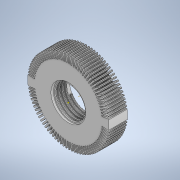
# Autodesk Inventor part: Scheibe
Saved by Autodesk Inventor 2020 (Build 240168000, 168)
## iProperties
Created: 2019-06-20
Part Number: Scheibe
Material: Generisch
Document SubType Name: Modeling
Designer: Limmer
Density: 1 g/cm^3
Appearance: Vorgabe
Author: Limmer
Autodesk Inventor part; units mm, degrees
(part 1 of 2)
ref_plane "YZ Plane" through (0, 0, 0) normal (1, 0, 0) x (0, 1, 0)
ref_plane "XZ Plane" through (0, 0, 0) normal (0, 1, 0) x (-1, 0, 0)
ref_plane "XY Plane" through (0, 0, 0) normal (0, 0, 1) x (1, 0, 0)
sketch "Skizze1" plane through (0, 0, 0) normal (0, 0, 1) x (1, 0, 0)
  circle A0 centre (0, 0) radius 17.5
  circle A1 centre (0, 0) radius 7.5
  dimension "d0" = 35
  dimension "d1" = 15
  constraints: 2 centre point, 2 coincident
  measures "d0" diameter of A0
  measures "d1" diameter of A1
extrude "Extrusion1" add sketch "Skizze1" along normal blind 8
sketch "Skizze2" plane through (0, 0, 0) normal (1, 0, 0) x (0, 1, 0)
  line L0 (-7.5, 0) -> (7.5, 0) projected
  line L1 (-7.5, 8) -> (7.5, 8) projected
  line L2 (7.5, 8) -> (6.75, 8)
  line L3 (6.75, 8) -> (6.75, 7.25)
  line L4 (6.75, 7.25) -> (7.5, 7.25)
  line L5 (7.5, 7.25) -> (7.5, 8)
  point P0 (0, 0)
  dimension "d4" = 0.75
  dimension "d5" = 0.75
  constraints: 8 end point, 2 parallel, 1 horizontal, 1 perpendicular
  measures "d4" distance of L4.end L3.end
  measures "d5" distance of L3.end L2.end
coil "Spirale1" sketch "Skizze2" operation add axis through (0, 0, 0) along (0, 0, -1) pitch 1.5 turns 4.666667 hand right
fillet "Rundung1" radius 0.25 20 edges at (2.7455, -6.1664, 1.35) (6.713, 0.7056, 7.65) (5.8457, 3.375, 6.25) (-6.4196, -2.0859, 6.95) (-1.4034, 6.6025, 2.05) (0, -6.75, 2.75) (1.4034, 6.6025, 3.45) (-5.0162, -4.5166, 5.55) (3.9676, 5.4609, 4.85) (-2.7455, -6.1664, 4.15) (2.7455, -6.1664, 0.6) (1.4034, 6.6025, 2.7) (0, -6.75, 2) (-1.4034, 6.6025, 1.3) (6.713, 0.7056, 6.9) (3.9676, 5.4609, 4.1) (-2.7455, -6.1664, 3.4) (5.8457, 3.375, 5.5) (-6.4196, -2.0859, 6.2) (-5.0162, -4.5166, 4.8)
fillet "Rundung2" radius 0.25 10 edges at (0, 6.75, 7.625) (0, 6.8232, 7.3233) (0, 7.25, 7.25) (0, 7.25, 8) (0, 6.8232, 7.9267) (-6.2787, -3.625, 1) (-5.8457, -3.375, 0.625) (-5.9091, -3.4116, 0.3233) (-6.2787, -3.625, 0.25) (-5.9091, -3.4116, 0.9267)
sketch "Skizze4" plane through (0, 0, 8) normal (0, 0, 1) x (1, 0, 0)
  point P0 (0, 0)
sketch "Skizze5" plane through (0, 0, 8) normal (0, 0, 1) x (1, 0, 0)
  circle A0 centre (0, 0) radius 17.5 projected
  line L0 (0, -17.2583) -> (0, -14.738)
  line L1 (0, 0) -> (-0.506, -14.4912) construction
  line L2 (0, 0) -> (0, -17) construction
  arc A1 (0.2433, -17.4983) -> (0.3675, -17.4961) centre (0, 0) ccw
  line L3 (0.5147, -14.7379) -> (0.6023, -17.2478) construction
  line L4 (0, 0) -> (0, -17.5) construction
  line L5 (0.5147, -14.7379) -> (0.6023, -17.2478)
  arc A2 (0.7422, -14.4898) -> (0.7764, -14.488) centre (0, 0) ccw
  line L6 (0, 0) -> (1.0121, -14.4735) construction
  line L7 (0, 0) -> (0.5064, -14.5) construction
  arc A3 (0, -17.2583) -> (0.2433, -17.4983) centre (0.24, -17.2583) ccw
  arc A4 (0.3675, -17.4961) -> (0.6023, -17.2478) centre (0.3625, -17.2562) ccw
  arc A5 (0.7422, -14.4898) -> (0.5147, -14.7379) centre (0.7545, -14.7295) ccw
  arc A6 (1.0287, -14.711) -> (0.7764, -14.488) centre (0.7893, -14.7277) ccw
  arc A7 (1.2039, -17.2163) -> (1.4634, -17.4387) centre (1.4433, -17.1995) ccw
  arc A8 (1.4634, -17.4387) -> (1.5871, -17.4279) centre (0, 0) ccw
  arc A9 (1.5871, -17.4279) -> (1.804, -17.1638) centre (1.5653, -17.1889) ccw
  arc A10 (1.7512, -14.4028) -> (1.5415, -14.6661) centre (1.7802, -14.641) ccw
  line L8 (1.5415, -14.6661) -> (1.804, -17.1638)
  arc A11 (2.0524, -14.6034) -> (1.7852, -14.3986) centre (1.8147, -14.6368) ccw
  arc A12 (1.7512, -14.4028) -> (1.7852, -14.3986) centre (0, 0) ccw
  line L9 (0, 0) -> (1.2207, -17.4574) construction
  line L10 (1.2039, -17.2163) -> (1.0281, -14.7021)
  arc A13 (2.4019, -17.0904) -> (2.6763, -17.2941) centre (2.6396, -17.057) ccw
  arc A14 (2.6763, -17.2941) -> (2.7989, -17.2747) centre (0, 0) ccw
  arc A15 (2.7989, -17.2747) -> (2.9969, -16.9961) centre (2.7605, -17.0378) ccw
  arc A16 (2.7516, -14.2455) -> (2.5608, -14.5228) centre (2.7971, -14.4812) ccw
  line L11 (2.5608, -14.5228) -> (2.9969, -16.9961)
  arc A17 (3.066, -14.4246) -> (2.7852, -14.239) centre (2.8313, -14.4745) ccw
  arc A18 (2.7516, -14.2455) -> (2.7852, -14.239) centre (0, 0) ccw
  line L12 (0, 0) -> (2.4355, -17.3297) construction
  line L13 (2.4019, -17.0904) -> (2.0511, -14.5946)
  arc A19 (3.5882, -16.8812) -> (3.8761, -17.0653) centre (3.823, -16.8313) ccw
  arc A20 (3.8761, -17.0653) -> (3.9971, -17.0374) centre (0, 0) ccw
  arc A21 (3.9971, -17.0374) -> (4.1752, -16.7457) centre (3.9423, -16.8037) ccw
  arc A22 (3.7386, -14.0189) -> (3.5676, -14.3088) centre (3.8005, -14.2508) ccw
  line L14 (3.5676, -14.3088) -> (4.1752, -16.7457)
  arc A23 (4.0648, -14.1756) -> (3.7717, -14.01) centre (3.8341, -14.2418) ccw
  arc A24 (3.7386, -14.0189) -> (3.7717, -14.01) centre (0, 0) ccw
  line L15 (0, 0) -> (3.6385, -17.1176) construction
  line L16 (3.5882, -16.8812) -> (3.0642, -14.416)
  arc A25 (4.757, -16.5898) -> (5.0571, -16.7534) centre (4.9877, -16.5236) ccw
  arc A26 (5.0571, -16.7534) -> (5.1758, -16.7171) centre (0, 0) ccw
  arc A27 (5.1758, -16.7171) -> (5.3331, -16.4136) centre (5.1049, -16.4878) ccw
  arc A28 (4.7074, -13.7239) -> (4.557, -14.0251) centre (4.7853, -13.951) ccw
  line L17 (4.557, -14.0251) -> (5.3331, -16.4136)
  arc A29 (5.0437, -13.8575) -> (4.7398, -13.7128) centre (4.8182, -13.9396) ccw
  arc A30 (4.7074, -13.7239) -> (4.7398, -13.7128) centre (0, 0) ccw
  line L18 (0, 0) -> (4.8237, -16.8221) construction
  line L19 (4.757, -16.5898) -> (4.0624, -14.1671)
  arc A31 (5.9027, -16.2175) -> (6.2134, -16.3598) centre (6.1282, -16.1354) ccw
  arc A32 (6.2134, -16.3598) -> (6.3294, -16.3153) centre (0, 0) ccw
  arc A33 (6.3294, -16.3153) -> (6.4651, -16.0016) centre (6.2426, -16.0916) ccw
  arc A34 (5.6533, -13.3621) -> (5.5243, -13.6731) centre (5.7468, -13.5832) ccw
  line L20 (5.5243, -13.6731) -> (6.4651, -16.0016)
  arc A35 (5.9981, -13.472) -> (5.6848, -13.3488) centre (5.7788, -13.5696) ccw
  arc A36 (5.6533, -13.3621) -> (5.6848, -13.3488) centre (0, 0) ccw
  line L21 (0, 0) -> (5.9854, -16.4446) construction
  line L22 (5.9027, -16.2175) -> (5.0407, -13.8492)
  arc A37 (7.0196, -15.7663) -> (7.3395, -15.8865) centre (7.2388, -15.6687) ccw
  arc A38 (7.3395, -15.8865) -> (7.452, -15.834) centre (0, 0) ccw
  arc A39 (7.452, -15.834) -> (7.5656, -15.5117) centre (7.3498, -15.6169) ccw
  arc A40 (6.5716, -12.9352) -> (6.4646, -13.2544) centre (6.6803, -13.1492) ccw
  line L23 (6.4646, -13.2544) -> (7.5656, -15.5117)
  arc A41 (6.9232, -13.0207) -> (6.6021, -12.9197) centre (6.7113, -13.1334) ccw
  arc A42 (6.5716, -12.9352) -> (6.6021, -12.9197) centre (0, 0) ccw
  line L24 (0, 0) -> (7.1179, -15.987) construction
  line L25 (7.0196, -15.7663) -> (5.9945, -13.4639)
  arc A43 (8.1023, -15.2382) -> (8.4298, -15.3358) centre (8.3142, -15.1255) ccw
  arc A44 (8.4298, -15.3358) -> (8.5384, -15.2756) centre (0, 0) ccw
  arc A45 (8.5384, -15.2756) -> (8.6292, -14.9462) centre (8.4213, -15.0662) ccw
  arc A46 (7.4579, -12.4453) -> (7.3734, -12.7712) centre (7.5813, -12.6512) ccw
  line L26 (7.3734, -12.7712) -> (8.6292, -14.9462)
  arc A47 (7.8147, -12.5061) -> (7.4873, -12.4277) centre (7.6111, -12.6332) ccw
  arc A48 (7.4579, -12.4453) -> (7.4873, -12.4277) centre (0, 0) ccw
  line L27 (0, 0) -> (8.2158, -15.4516) construction
  line L28 (8.1023, -15.2382) -> (6.9191, -13.0129)
  arc A49 (9.1455, -14.6359) -> (9.4791, -14.7105) centre (9.3491, -14.5087) ccw
  arc A50 (9.4791, -14.7105) -> (9.5832, -14.6428) centre (0, 0) ccw
  arc A51 (9.5832, -14.6428) -> (9.6507, -14.3078) centre (9.4518, -14.442) ccw
  arc A52 (8.3079, -11.8948) -> (8.2464, -12.2257) centre (8.4453, -12.0915) ccw
  line L29 (8.2464, -12.2257) -> (9.6507, -14.3078)
  arc A53 (8.668, -11.9305) -> (8.3359, -11.8751) centre (8.4738, -12.0715) ccw
  arc A54 (8.3079, -11.8948) -> (8.3359, -11.8751) centre (0, 0) ccw
  line L30 (0, 0) -> (9.2736, -14.8408) construction
  line L31 (9.1455, -14.6359) -> (7.81, -12.4986)
  arc A55 (10.1442, -13.9623) -> (10.4821, -14.0134) centre (10.3384, -13.8212) ccw
  arc A56 (10.4821, -14.0134) -> (10.5813, -13.9387) centre (0, 0) ccw
  arc A57 (10.5813, -13.9387) -> (10.6253, -13.5998) centre (10.4362, -13.7475) ccw
  arc A58 (9.1174, -11.2863) -> (9.0791, -11.6207) centre (9.2682, -11.4729) ccw
  line L32 (9.0791, -11.6207) -> (10.6253, -13.5998)
  arc A59 (9.4791, -11.2968) -> (9.144, -11.2647) centre (9.2953, -11.451) ccw
  arc A60 (9.1174, -11.2863) -> (9.144, -11.2647) centre (0, 0) ccw
  line L33 (0, 0) -> (10.2862, -14.1578) construction
  line L34 (10.1442, -13.9623) -> (8.6628, -11.9233)
  arc A61 (11.0934, -13.2206) -> (11.4341, -13.2481) centre (11.2773, -13.0664) ccw
  arc A62 (11.4341, -13.2481) -> (11.5278, -13.1666) centre (0, 0) ccw
  arc A63 (11.5278, -13.1666) -> (11.5481, -12.8254) centre (11.3697, -12.986) ccw
  arc A64 (9.8825, -10.6228) -> (9.8676, -10.9591) centre (10.0459, -10.7985) ccw
  line L35 (9.8676, -10.9591) -> (11.5481, -12.8254)
  arc A65 (10.244, -10.608) -> (9.9075, -10.5994) centre (10.0714, -10.7747) ccw
  arc A66 (9.8825, -10.6228) -> (9.9075, -10.5994) centre (0, 0) ccw
  line L36 (0, 0) -> (11.2488, -13.4058) construction
  line L37 (11.0934, -13.2206) -> (9.4734, -11.29)
  arc A67 (11.9886, -12.4146) -> (12.3304, -12.4182) centre (12.1613, -12.2479) ccw
  arc A68 (12.3304, -12.4182) -> (12.4182, -12.3304) centre (0, 0) ccw
  arc A69 (12.4182, -12.3304) -> (12.4146, -11.9886) centre (12.2479, -12.1613) ccw
  arc A70 (10.5994, -9.9075) -> (10.608, -10.244) centre (10.7747, -10.0714) ccw
  line L38 (10.608, -10.244) -> (12.4146, -11.9886)
  arc A71 (10.9591, -9.8676) -> (10.6228, -9.8825) centre (10.7985, -10.0459) ccw
  arc A72 (10.5994, -9.9075) -> (10.6228, -9.8825) centre (0, 0) ccw
  line L39 (0, 0) -> (12.1565, -12.5884) construction
  line L40 (11.9886, -12.4146) -> (10.2379, -10.6017)
  arc A73 (12.8254, -11.5481) -> (13.1666, -11.5278) centre (12.986, -11.3697) ccw
  arc A74 (13.1666, -11.5278) -> (13.2481, -11.4341) centre (0, 0) ccw
  arc A75 (13.2481, -11.4341) -> (13.2206, -11.0934) centre (13.0664, -11.2773) ccw
  arc A76 (11.2647, -9.144) -> (11.2968, -9.4791) centre (11.451, -9.2953) ccw
  line L41 (11.2968, -9.4791) -> (13.2206, -11.0934)
  arc A77 (11.6207, -9.0791) -> (11.2863, -9.1174) centre (11.4729, -9.2682) ccw
  arc A78 (11.2647, -9.144) -> (11.2863, -9.1174) centre (0, 0) ccw
  line L42 (0, 0) -> (13.005, -11.7098) construction
  line L43 (12.8254, -11.5481) -> (10.9525, -9.8617)
  arc A79 (13.5998, -10.6253) -> (13.9387, -10.5813) centre (13.7475, -10.4362) ccw
  arc A80 (13.9387, -10.5813) -> (14.0134, -10.4821) centre (0, 0) ccw
  arc A81 (14.0134, -10.4821) -> (13.9623, -10.1442) centre (13.8212, -10.3384) ccw
  arc A82 (11.8751, -8.3359) -> (11.9305, -8.668) centre (12.0715, -8.4738) ccw
  line L44 (11.9305, -8.668) -> (13.9623, -10.1442)
  arc A83 (12.2257, -8.2464) -> (11.8948, -8.3079) centre (12.0915, -8.4453) ccw
  arc A84 (11.8751, -8.3359) -> (11.8948, -8.3079) centre (0, 0) ccw
  line L45 (0, 0) -> (13.7902, -10.7741) construction
  line L46 (13.5998, -10.6253) -> (11.6137, -9.0736)
  arc A85 (14.3078, -9.6507) -> (14.6428, -9.5832) centre (14.442, -9.4518) ccw
  arc A86 (14.6428, -9.5832) -> (14.7105, -9.4791) centre (0, 0) ccw
  arc A87 (14.7105, -9.4791) -> (14.6359, -9.1455) centre (14.5087, -9.3491) ccw
  arc A88 (12.4277, -7.4873) -> (12.5061, -7.8147) centre (12.6332, -7.6111) ccw
  line L47 (12.5061, -7.8147) -> (14.6359, -9.1455)
  arc A89 (12.7712, -7.3734) -> (12.4453, -7.4579) centre (12.6512, -7.5813) ccw
  arc A90 (12.4277, -7.4873) -> (12.4453, -7.4579) centre (0, 0) ccw
  line L48 (0, 0) -> (14.5082, -9.7859) construction
  line L49 (14.3078, -9.6507) -> (12.2184, -8.2414)
  arc A91 (14.9462, -8.6292) -> (15.2756, -8.5384) centre (15.0662, -8.4213) ccw
  arc A92 (15.2756, -8.5384) -> (15.3358, -8.4298) centre (0, 0) ccw
  arc A93 (15.3358, -8.4298) -> (15.2382, -8.1023) centre (15.1255, -8.3142) ccw
  arc A94 (12.9197, -6.6021) -> (13.0207, -6.9232) centre (13.1334, -6.7113) ccw
  line L50 (13.0207, -6.9232) -> (15.2382, -8.1023)
  arc A95 (13.2544, -6.4646) -> (12.9352, -6.5716) centre (13.1492, -6.6803) ccw
  arc A96 (12.9197, -6.6021) -> (12.9352, -6.5716) centre (0, 0) ccw
  line L51 (0, 0) -> (15.1554, -8.75) construction
  line L52 (14.9462, -8.6292) -> (12.7635, -7.369)
  arc A97 (15.5117, -7.5656) -> (15.834, -7.452) centre (15.6169, -7.3498) ccw
  arc A98 (15.834, -7.452) -> (15.8865, -7.3395) centre (0, 0) ccw
  arc A99 (15.8865, -7.3395) -> (15.7663, -7.0196) centre (15.6687, -7.2388) ccw
  arc A100 (13.3488, -5.6848) -> (13.472, -5.9981) centre (13.5696, -5.7788) ccw
  line L53 (13.472, -5.9981) -> (15.7663, -7.0196)
  arc A101 (13.6731, -5.5243) -> (13.3621, -5.6533) centre (13.5832, -5.7468) ccw
  arc A102 (13.3488, -5.6848) -> (13.3621, -5.6533) centre (0, 0) ccw
  line L54 (0, 0) -> (15.7289, -7.6715) construction
  line L55 (15.5117, -7.5656) -> (13.2465, -6.4607)
  arc A103 (16.0016, -6.4651) -> (16.3153, -6.3294) centre (16.0916, -6.2426) ccw
  arc A104 (16.3153, -6.3294) -> (16.3598, -6.2134) centre (0, 0) ccw
  arc A105 (16.3598, -6.2134) -> (16.2175, -5.9027) centre (16.1354, -6.1282) ccw
  arc A106 (13.7128, -4.7398) -> (13.8575, -5.0437) centre (13.9396, -4.8182) ccw
  line L56 (13.8575, -5.0437) -> (16.2175, -5.9027)
  arc A107 (14.0251, -4.557) -> (13.7239, -4.7074) centre (13.951, -4.7853) ccw
  arc A108 (13.7128, -4.7398) -> (13.7239, -4.7074) centre (0, 0) ccw
  line L57 (0, 0) -> (16.2257, -6.5556) construction
  line L58 (16.0016, -6.4651) -> (13.6649, -5.521)
  arc A109 (16.4136, -5.3331) -> (16.7171, -5.1758) centre (16.4878, -5.1049) ccw
  arc A110 (16.7171, -5.1758) -> (16.7534, -5.0571) centre (0, 0) ccw
  arc A111 (16.7534, -5.0571) -> (16.5898, -4.757) centre (16.5236, -4.9877) ccw
  arc A112 (14.01, -3.7717) -> (14.1756, -4.0648) centre (14.2418, -3.8341) ccw
  line L59 (14.1756, -4.0648) -> (16.5898, -4.757)
  arc A113 (14.3088, -3.5676) -> (14.0189, -3.7386) centre (14.2508, -3.8005) ccw
  arc A114 (14.01, -3.7717) -> (14.0189, -3.7386) centre (0, 0) ccw
  line L60 (0, 0) -> (16.6435, -5.4078) construction
  line L61 (16.4136, -5.3331) -> (14.0167, -4.5543)
  arc A115 (16.7457, -4.1752) -> (17.0374, -3.9971) centre (16.8037, -3.9423) ccw
  arc A116 (17.0374, -3.9971) -> (17.0653, -3.8761) centre (0, 0) ccw
  arc A117 (17.0653, -3.8761) -> (16.8812, -3.5882) centre (16.8313, -3.823) ccw
  arc A118 (14.239, -2.7852) -> (14.4246, -3.066) centre (14.4745, -2.8313) ccw
  line L62 (14.4246, -3.066) -> (16.8812, -3.5882)
  arc A119 (14.5228, -2.5608) -> (14.2455, -2.7516) centre (14.4812, -2.7971) ccw
  arc A120 (14.239, -2.7852) -> (14.2455, -2.7516) centre (0, 0) ccw
  line L63 (0, 0) -> (16.9802, -4.2336) construction
  line L64 (16.7457, -4.1752) -> (14.3003, -3.5655)
  arc A121 (16.9961, -2.9969) -> (17.2747, -2.7989) centre (17.0378, -2.7605) ccw
  arc A122 (17.2747, -2.7989) -> (17.2941, -2.6763) centre (0, 0) ccw
  arc A123 (17.2941, -2.6763) -> (17.0904, -2.4019) centre (17.057, -2.6396) ccw
  arc A124 (14.3986, -1.7852) -> (14.6034, -2.0524) centre (14.6368, -1.8147) ccw
  line L65 (14.6034, -2.0524) -> (17.0904, -2.4019)
  arc A125 (14.6661, -1.5415) -> (14.4028, -1.7512) centre (14.641, -1.7802) ccw
  arc A126 (14.3986, -1.7852) -> (14.4028, -1.7512) centre (0, 0) ccw
  line L66 (0, 0) -> (17.2341, -3.0388) construction
  line L67 (16.9961, -2.9969) -> (14.5141, -2.5592)
  arc A127 (17.1638, -1.804) -> (17.4279, -1.5871) centre (17.1889, -1.5653) ccw
  arc A128 (17.4279, -1.5871) -> (17.4387, -1.4634) centre (0, 0) ccw
  arc A129 (17.4387, -1.4634) -> (17.2163, -1.2039) centre (17.1995, -1.4433) ccw
  arc A130 (14.488, -0.7764) -> (14.711, -1.0287) centre (14.7277, -0.7893) ccw
  line L68 (14.711, -1.0287) -> (17.2163, -1.2039)
  arc A131 (14.7379, -0.5147) -> (14.4898, -0.7422) centre (14.7295, -0.7545) ccw
  arc A132 (14.488, -0.7764) -> (14.4898, -0.7422) centre (0, 0) ccw
  line L69 (0, 0) -> (17.4041, -1.8292) construction
  line L70 (17.1638, -1.804) -> (14.6573, -1.5405)
  arc A133 (17.2478, -0.6023) -> (17.4961, -0.3675) centre (17.2562, -0.3625) ccw
  arc A134 (17.4961, -0.3675) -> (17.4983, -0.2433) centre (0, 0) ccw
  arc A135 (17.4983, -0.2433) -> (17.2583, 0) centre (17.2583, -0.24) ccw
  arc A136 (14.5069, 0.2361) -> (14.7469, 0) centre (14.7469, 0.24) ccw
  line L71 (14.7469, 0) -> (17.2583, 0)
  arc A137 (14.7379, 0.5147) -> (14.5063, 0.2703) centre (14.7463, 0.2748) ccw
  arc A138 (14.5069, 0.2361) -> (14.5063, 0.2703) centre (0, 0) ccw
  line L72 (0, 0) -> (17.4893, -0.6107) construction
  line L73 (17.2478, -0.6023) -> (14.7291, -0.5144)
  arc A139 (17.2478, 0.6023) -> (17.4792, 0.8539) centre (17.2394, 0.8422) ccw
  arc A140 (17.4792, 0.8539) -> (17.4727, 0.9779) centre (0, 0) ccw
  arc A141 (17.4727, 0.9779) -> (17.2163, 1.2039) centre (17.233, 0.9645) ccw
  arc A142 (14.4551, 1.2475) -> (14.711, 1.0287) centre (14.6942, 1.2681) ccw
  line L74 (14.711, 1.0287) -> (17.2163, 1.2039)
  arc A143 (14.6661, 1.5415) -> (14.4521, 1.2816) centre (14.6912, 1.3028) ccw
  arc A144 (14.4551, 1.2475) -> (14.4521, 1.2816) centre (0, 0) ccw
  line L75 (0, 0) -> (17.4893, 0.6107) construction
  line L76 (17.2478, 0.6023) -> (14.7291, 0.5144)
  arc A145 (17.1638, 1.804) -> (17.377, 2.0711) centre (17.1387, 2.0427) ccw
  arc A146 (17.377, 2.0711) -> (17.3619, 2.1943) centre (0, 0) ccw
  arc A147 (17.3619, 2.1943) -> (17.0904, 2.4019) centre (17.1238, 2.1642) ccw
  arc A148 (14.3329, 2.2528) -> (14.6034, 2.0524) centre (14.57, 2.29) ccw
  line L77 (14.6034, 2.0524) -> (17.0904, 2.4019)
  arc A149 (14.5228, 2.5608) -> (14.3275, 2.2866) centre (14.5645, 2.3244) ccw
  arc A150 (14.3329, 2.2528) -> (14.3275, 2.2866) centre (0, 0) ccw
  line L78 (0, 0) -> (17.4041, 1.8292) construction
  line L79 (17.1638, 1.804) -> (14.6573, 1.5405)
  arc A151 (16.9961, 2.9969) -> (17.1902, 3.2782) centre (16.9545, 3.2332) ccw
  arc A152 (17.1902, 3.2782) -> (17.1665, 3.4001) centre (0, 0) ccw
  arc A153 (17.1665, 3.4001) -> (16.8812, 3.5882) centre (16.9311, 3.3535) ccw
  arc A154 (14.1408, 3.2471) -> (14.4246, 3.066) centre (14.3747, 3.3008) ccw
  line L80 (14.4246, 3.066) -> (16.8812, 3.5882)
  arc A155 (14.3088, 3.5676) -> (14.1331, 3.2805) centre (14.3669, 3.3347) ccw
  arc A156 (14.1408, 3.2471) -> (14.1331, 3.2805) centre (0, 0) ccw
  line L81 (0, 0) -> (17.2341, 3.0388) construction
  line L82 (16.9961, 2.9969) -> (14.5141, 2.5592)
  arc A157 (16.7457, 4.1752) -> (16.9197, 4.4693) centre (16.6876, 4.408) ccw
  arc A158 (16.9197, 4.4693) -> (16.8875, 4.5893) centre (0, 0) ccw
  arc A159 (16.8875, 4.5893) -> (16.5898, 4.757) centre (16.6559, 4.5263) ccw
  arc A160 (13.8799, 4.2256) -> (14.1756, 4.0648) centre (14.1095, 4.2955) ccw
  line L83 (14.1756, 4.0648) -> (16.5898, 4.757)
  arc A161 (14.0251, 4.557) -> (13.8699, 4.2583) centre (14.0993, 4.3288) ccw
  arc A162 (13.8799, 4.2256) -> (13.8699, 4.2583) centre (0, 0) ccw
  line L84 (0, 0) -> (16.9802, 4.2336) construction
  line L85 (16.7457, 4.1752) -> (14.3003, 3.5655)
  arc A163 (16.4136, 5.3331) -> (16.5667, 5.6387) centre (16.3395, 5.5614) ccw
  arc A164 (16.5667, 5.6387) -> (16.5263, 5.7561) centre (0, 0) ccw
  arc A165 (16.5263, 5.7561) -> (16.2175, 5.9027) centre (16.2996, 5.6772) ccw
  arc A166 (13.5513, 5.1835) -> (13.8575, 5.0437) centre (13.7755, 5.2693) ccw
  line L86 (13.8575, 5.0437) -> (16.2175, 5.9027)
  arc A167 (13.6731, 5.5243) -> (13.539, 5.2155) centre (13.763, 5.3018) ccw
  arc A168 (13.5513, 5.1835) -> (13.539, 5.2155) centre (0, 0) ccw
  line L87 (0, 0) -> (16.6435, 5.4078) construction
  line L88 (16.4136, 5.3331) -> (14.0167, 4.5543)
  arc A169 (16.0016, 6.4651) -> (16.133, 6.7806) centre (15.9117, 6.6876) ccw
  arc A170 (16.133, 6.7806) -> (16.0845, 6.8949) centre (0, 0) ccw
  arc A171 (16.0845, 6.8949) -> (15.7663, 7.0196) centre (15.8639, 6.8003) ccw
  arc A172 (13.1567, 6.1162) -> (13.472, 5.9981) centre (13.3743, 6.2173) ccw
  line L89 (13.472, 5.9981) -> (15.7663, 7.0196)
  arc A173 (13.2544, 6.4646) -> (13.1422, 6.1472) centre (13.3596, 6.2489) ccw
  arc A174 (13.1567, 6.1162) -> (13.1422, 6.1472) centre (0, 0) ccw
  line L90 (0, 0) -> (16.2257, 6.5556) construction
  line L91 (16.0016, 6.4651) -> (13.6649, 5.521)
  arc A175 (15.5117, 7.5656) -> (15.6207, 7.8895) centre (15.4065, 7.7813) ccw
  arc A176 (15.6207, 7.8895) -> (15.5643, 8.0001) centre (0, 0) ccw
  arc A177 (15.5643, 8.0001) -> (15.2382, 8.1023) centre (15.3509, 7.8904) ccw
  arc A178 (12.698, 7.019) -> (13.0207, 6.9232) centre (12.9081, 7.1352) ccw
  line L92 (13.0207, 6.9232) -> (15.2382, 8.1023)
  arc A179 (12.7712, 7.3734) -> (12.6814, 7.049) centre (12.8912, 7.1656) ccw
  arc A180 (12.698, 7.019) -> (12.6814, 7.049) centre (0, 0) ccw
  line L93 (0, 0) -> (15.7289, 7.6715) construction
  line L94 (15.5117, 7.5656) -> (13.2465, 6.4607)
  arc A181 (14.9462, 8.6292) -> (15.0323, 8.9599) centre (14.8262, 8.837) ccw
  arc A182 (15.0323, 8.9599) -> (14.9684, 9.0663) centre (0, 0) ccw
  arc A183 (14.9684, 9.0663) -> (14.6359, 9.1455) centre (14.7631, 8.942) ccw
  arc A184 (12.1775, 7.8877) -> (12.5061, 7.8147) centre (12.3789, 8.0182) ccw
  line L95 (12.5061, 7.8147) -> (14.6359, 9.1455)
  arc A185 (12.2257, 8.2464) -> (12.1588, 7.9164) centre (12.3599, 8.0474) ccw
  arc A186 (12.1775, 7.8877) -> (12.1588, 7.9164) centre (0, 0) ccw
  line L96 (0, 0) -> (15.1554, 8.75) construction
  line L97 (14.9462, 8.6292) -> (12.7635, 7.369)
  arc A187 (14.3078, 9.6507) -> (14.3707, 9.9867) centre (14.1736, 9.8497) ccw
  arc A188 (14.3707, 9.9867) -> (14.2995, 10.0884) centre (0, 0) ccw
  arc A189 (14.2995, 10.0884) -> (13.9623, 10.1442) centre (14.1034, 9.95) ccw
  arc A190 (11.5976, 8.718) -> (11.9305, 8.668) centre (11.7894, 8.8622) ccw
  line L98 (11.9305, 8.668) -> (13.9623, 10.1442)
  arc A191 (11.6207, 9.0791) -> (11.577, 8.7453) centre (11.7685, 8.89) ccw
  arc A192 (11.5976, 8.718) -> (11.577, 8.7453) centre (0, 0) ccw
  line L99 (0, 0) -> (14.5082, 9.7859) construction
  line L100 (14.3078, 9.6507) -> (12.2184, 8.2414)
  arc A193 (13.5998, 10.6253) -> (13.639, 10.9648) centre (13.452, 10.8144) ccw
  arc A194 (13.639, 10.9648) -> (13.5609, 11.0613) centre (0, 0) ccw
  arc A195 (13.5609, 11.0613) -> (13.2206, 11.0934) centre (13.3749, 10.9096) ccw
  arc A196 (10.9612, 9.5057) -> (11.2968, 9.4791) centre (11.1425, 9.663) ccw
  line L101 (11.2968, 9.4791) -> (13.2206, 11.0934)
  arc A197 (10.9591, 9.8676) -> (10.9387, 9.5316) centre (11.1197, 9.6892) ccw
  arc A198 (10.9612, 9.5057) -> (10.9387, 9.5316) centre (0, 0) ccw
  line L102 (0, 0) -> (13.7902, 10.7741) construction
  line L103 (13.5998, 10.6253) -> (11.6137, 9.0736)
  arc A199 (12.8254, 11.5481) -> (12.841, 11.8895) centre (12.6648, 11.7264) ccw
  arc A200 (12.841, 11.8895) -> (12.7563, 11.9803) centre (0, 0) ccw
  arc A201 (12.7563, 11.9803) -> (12.4146, 11.9886) centre (12.5813, 11.816) ccw
  arc A202 (10.2714, 10.2472) -> (10.608, 10.244) centre (10.4413, 10.4167) ccw
  line L104 (10.608, 10.244) -> (12.4146, 11.9886)
  arc A203 (10.244, 10.608) -> (10.2472, 10.2714) centre (10.4167, 10.4413) ccw
  arc A204 (10.2714, 10.2472) -> (10.2472, 10.2714) centre (0, 0) ccw
  line L105 (0, 0) -> (13.005, 11.7098) construction
  line L106 (12.8254, 11.5481) -> (10.9525, 9.8617)
  arc A205 (11.9886, 12.4146) -> (11.9803, 12.7563) centre (11.816, 12.5813) ccw
  arc A206 (11.9803, 12.7563) -> (11.8895, 12.841) centre (0, 0) ccw
  arc A207 (11.8895, 12.841) -> (11.5481, 12.8254) centre (11.7264, 12.6648) ccw
  arc A208 (9.5316, 10.9387) -> (9.8676, 10.9591) centre (9.6892, 11.1197) ccw
  line L107 (9.8676, 10.9591) -> (11.5481, 12.8254)
  arc A209 (9.4791, 11.2968) -> (9.5057, 10.9612) centre (9.663, 11.1425) ccw
  arc A210 (9.5316, 10.9387) -> (9.5057, 10.9612) centre (0, 0) ccw
  line L108 (0, 0) -> (12.1565, 12.5884) construction
  line L109 (11.9886, 12.4146) -> (10.2379, 10.6017)
  arc A211 (11.0934, 13.2206) -> (11.0613, 13.5609) centre (10.9096, 13.3749) ccw
  arc A212 (11.0613, 13.5609) -> (10.9648, 13.639) centre (0, 0) ccw
  arc A213 (10.9648, 13.639) -> (10.6253, 13.5998) centre (10.8144, 13.452) ccw
  arc A214 (8.7453, 11.577) -> (9.0791, 11.6207) centre (8.89, 11.7685) ccw
  line L110 (9.0791, 11.6207) -> (10.6253, 13.5998)
  arc A215 (8.668, 11.9305) -> (8.718, 11.5976) centre (8.8622, 11.7894) ccw
  arc A216 (8.7453, 11.577) -> (8.718, 11.5976) centre (0, 0) ccw
  line L111 (0, 0) -> (11.2488, 13.4058) construction
  line L112 (11.0934, 13.2206) -> (9.4734, 11.29)
  arc A217 (10.1442, 13.9623) -> (10.0884, 14.2995) centre (9.95, 14.1034) ccw
  arc A218 (10.0884, 14.2995) -> (9.9867, 14.3707) centre (0, 0) ccw
  arc A219 (9.9867, 14.3707) -> (9.6507, 14.3078) centre (9.8497, 14.1736) ccw
  arc A220 (7.9164, 12.1588) -> (8.2464, 12.2257) centre (8.0474, 12.3599) ccw
  line L113 (8.2464, 12.2257) -> (9.6507, 14.3078)
  arc A221 (7.8147, 12.5061) -> (7.8877, 12.1775) centre (8.0182, 12.3789) ccw
  arc A222 (7.9164, 12.1588) -> (7.8877, 12.1775) centre (0, 0) ccw
  line L114 (0, 0) -> (10.2862, 14.1578) construction
  line L115 (10.1442, 13.9623) -> (8.6628, 11.9233)
  arc A223 (9.1455, 14.6359) -> (9.0663, 14.9684) centre (8.942, 14.7631) ccw
  arc A224 (9.0663, 14.9684) -> (8.9599, 15.0323) centre (0, 0) ccw
  arc A225 (8.9599, 15.0323) -> (8.6292, 14.9462) centre (8.837, 14.8262) ccw
  arc A226 (7.049, 12.6814) -> (7.3734, 12.7712) centre (7.1656, 12.8912) ccw
  line L116 (7.3734, 12.7712) -> (8.6292, 14.9462)
  arc A227 (6.9232, 13.0207) -> (7.019, 12.698) centre (7.1352, 12.9081) ccw
  arc A228 (7.049, 12.6814) -> (7.019, 12.698) centre (0, 0) ccw
  line L117 (0, 0) -> (9.2736, 14.8408) construction
  line L118 (9.1455, 14.6359) -> (7.81, 12.4986)
  arc A229 (8.1023, 15.2382) -> (8.0001, 15.5643) centre (7.8904, 15.3509) ccw
  arc A230 (8.0001, 15.5643) -> (7.8895, 15.6207) centre (0, 0) ccw
  arc A231 (7.8895, 15.6207) -> (7.5656, 15.5117) centre (7.7813, 15.4065) ccw
  arc A232 (6.1472, 13.1422) -> (6.4646, 13.2544) centre (6.2489, 13.3596) ccw
  line L119 (6.4646, 13.2544) -> (7.5656, 15.5117)
  arc A233 (5.9981, 13.472) -> (6.1162, 13.1567) centre (6.2173, 13.3743) ccw
  arc A234 (6.1472, 13.1422) -> (6.1162, 13.1567) centre (0, 0) ccw
  line L120 (0, 0) -> (8.2158, 15.4516) construction
  line L121 (8.1023, 15.2382) -> (6.9191, 13.0129)
  arc A235 (7.0196, 15.7663) -> (6.8949, 16.0845) centre (6.8003, 15.8639) ccw
  arc A236 (6.8949, 16.0845) -> (6.7806, 16.133) centre (0, 0) ccw
  arc A237 (6.7806, 16.133) -> (6.4651, 16.0016) centre (6.6876, 15.9117) ccw
  arc A238 (5.2155, 13.539) -> (5.5243, 13.6731) centre (5.3018, 13.763) ccw
  line L122 (5.5243, 13.6731) -> (6.4651, 16.0016)
  arc A239 (5.0437, 13.8575) -> (5.1835, 13.5513) centre (5.2693, 13.7755) ccw
  arc A240 (5.2155, 13.539) -> (5.1835, 13.5513) centre (0, 0) ccw
  line L123 (0, 0) -> (7.1179, 15.987) construction
  line L124 (7.0196, 15.7663) -> (5.9945, 13.4639)
  arc A241 (5.9027, 16.2175) -> (5.7561, 16.5263) centre (5.6772, 16.2996) ccw
  arc A242 (5.7561, 16.5263) -> (5.6387, 16.5667) centre (0, 0) ccw
  arc A243 (5.6387, 16.5667) -> (5.3331, 16.4136) centre (5.5614, 16.3395) ccw
  arc A244 (4.2583, 13.8699) -> (4.557, 14.0251) centre (4.3288, 14.0993) ccw
  line L125 (4.557, 14.0251) -> (5.3331, 16.4136)
  arc A245 (4.0648, 14.1756) -> (4.2256, 13.8799) centre (4.2955, 14.1095) ccw
  arc A246 (4.2583, 13.8699) -> (4.2256, 13.8799) centre (0, 0) ccw
  line L126 (0, 0) -> (5.9854, 16.4446) construction
  line L127 (5.9027, 16.2175) -> (5.0407, 13.8492)
  arc A247 (4.757, 16.5898) -> (4.5893, 16.8875) centre (4.5263, 16.6559) ccw
  arc A248 (4.5893, 16.8875) -> (4.4693, 16.9197) centre (0, 0) ccw
  arc A249 (4.4693, 16.9197) -> (4.1752, 16.7457) centre (4.408, 16.6876) ccw
  arc A250 (3.2805, 14.1331) -> (3.5676, 14.3088) centre (3.3347, 14.3669) ccw
  line L128 (3.5676, 14.3088) -> (4.1752, 16.7457)
  arc A251 (3.066, 14.4246) -> (3.2471, 14.1408) centre (3.3008, 14.3747) ccw
  arc A252 (3.2805, 14.1331) -> (3.2471, 14.1408) centre (0, 0) ccw
  line L129 (0, 0) -> (4.8237, 16.8221) construction
  line L130 (4.757, 16.5898) -> (4.0624, 14.1671)
  arc A253 (3.5882, 16.8812) -> (3.4001, 17.1665) centre (3.3535, 16.9311) ccw
  arc A254 (3.4001, 17.1665) -> (3.2782, 17.1902) centre (0, 0) ccw
  arc A255 (3.2782, 17.1902) -> (2.9969, 16.9961) centre (3.2332, 16.9545) ccw
  arc A256 (2.2866, 14.3275) -> (2.5608, 14.5228) centre (2.3244, 14.5645) ccw
  line L131 (2.5608, 14.5228) -> (2.9969, 16.9961)
  arc A257 (2.0524, 14.6034) -> (2.2528, 14.3329) centre (2.29, 14.57) ccw
  arc A258 (2.2866, 14.3275) -> (2.2528, 14.3329) centre (0, 0) ccw
  line L132 (0, 0) -> (3.6385, 17.1176) construction
  line L133 (3.5882, 16.8812) -> (3.0642, 14.416)
  arc A259 (2.4019, 17.0904) -> (2.1943, 17.3619) centre (2.1642, 17.1238) ccw
  arc A260 (2.1943, 17.3619) -> (2.0711, 17.377) centre (0, 0) ccw
  arc A261 (2.0711, 17.377) -> (1.804, 17.1638) centre (2.0427, 17.1387) ccw
  arc A262 (1.2816, 14.4521) -> (1.5415, 14.6661) centre (1.3028, 14.6912) ccw
  line L134 (1.5415, 14.6661) -> (1.804, 17.1638)
  arc A263 (1.0287, 14.711) -> (1.2475, 14.4551) centre (1.2681, 14.6942) ccw
  arc A264 (1.2816, 14.4521) -> (1.2475, 14.4551) centre (0, 0) ccw
  line L135 (0, 0) -> (2.4355, 17.3297) construction
  line L136 (2.4019, 17.0904) -> (2.0511, 14.5946)
  arc A265 (1.2039, 17.2163) -> (0.9779, 17.4727) centre (0.9645, 17.233) ccw
  arc A266 (0.9779, 17.4727) -> (0.8539, 17.4792) centre (0, 0) ccw
  arc A267 (0.8539, 17.4792) -> (0.6023, 17.2478) centre (0.8422, 17.2394) ccw
  arc A268 (0.2703, 14.5063) -> (0.5147, 14.7379) centre (0.2748, 14.7463) ccw
  line L137 (0.5147, 14.7379) -> (0.6023, 17.2478)
  arc A269 (0, 14.7469) -> (0.2361, 14.5069) centre (0.24, 14.7469) ccw
  arc A270 (0.2703, 14.5063) -> (0.2361, 14.5069) centre (0, 0) ccw
  line L138 (0, 0) -> (1.2207, 17.4574) construction
  line L139 (1.2039, 17.2163) -> (1.0281, 14.7021)
  arc A271 (0, 17.2583) -> (-0.2433, 17.4983) centre (-0.24, 17.2583) ccw
  arc A272 (-0.2433, 17.4983) -> (-0.3675, 17.4961) centre (0, 0) ccw
  arc A273 (-0.3675, 17.4961) -> (-0.6023, 17.2478) centre (-0.3625, 17.2562) ccw
  arc A274 (-0.7422, 14.4898) -> (-0.5147, 14.7379) centre (-0.7545, 14.7295) ccw
  line L140 (-0.5147, 14.7379) -> (-0.6023, 17.2478)
  arc A275 (-1.0287, 14.711) -> (-0.7764, 14.488) centre (-0.7893, 14.7277) ccw
  arc A276 (-0.7422, 14.4898) -> (-0.7764, 14.488) centre (0, 0) ccw
  line L141 (0, 0) -> (0, 17.5) construction
  line L142 (0, 17.2583) -> (0, 14.738)
  arc A277 (-1.2039, 17.2163) -> (-1.4634, 17.4387) centre (-1.4433, 17.1995) ccw
  arc A278 (-1.4634, 17.4387) -> (-1.5871, 17.4279) centre (0, 0) ccw
  arc A279 (-1.5871, 17.4279) -> (-1.804, 17.1638) centre (-1.5653, 17.1889) ccw
  arc A280 (-1.7512, 14.4028) -> (-1.5415, 14.6661) centre (-1.7802, 14.641) ccw
  line L143 (-1.5415, 14.6661) -> (-1.804, 17.1638)
  arc A281 (-2.0524, 14.6034) -> (-1.7852, 14.3986) centre (-1.8147, 14.6368) ccw
  arc A282 (-1.7512, 14.4028) -> (-1.7852, 14.3986) centre (0, 0) ccw
  line L144 (0, 0) -> (-1.2207, 17.4574) construction
  line L145 (-1.2039, 17.2163) -> (-1.0281, 14.7021)
  arc A283 (-2.4019, 17.0904) -> (-2.6763, 17.2941) centre (-2.6396, 17.057) ccw
  arc A284 (-2.6763, 17.2941) -> (-2.7989, 17.2747) centre (0, 0) ccw
  arc A285 (-2.7989, 17.2747) -> (-2.9969, 16.9961) centre (-2.7605, 17.0378) ccw
  arc A286 (-2.7516, 14.2455) -> (-2.5608, 14.5228) centre (-2.7971, 14.4812) ccw
  line L146 (-2.5608, 14.5228) -> (-2.9969, 16.9961)
  arc A287 (-3.066, 14.4246) -> (-2.7852, 14.239) centre (-2.8313, 14.4745) ccw
  arc A288 (-2.7516, 14.2455) -> (-2.7852, 14.239) centre (0, 0) ccw
  line L147 (0, 0) -> (-2.4355, 17.3297) construction
  line L148 (-2.4019, 17.0904) -> (-2.0511, 14.5946)
  arc A289 (-3.5882, 16.8812) -> (-3.8761, 17.0653) centre (-3.823, 16.8313) ccw
  arc A290 (-3.8761, 17.0653) -> (-3.9971, 17.0374) centre (0, 0) ccw
  arc A291 (-3.9971, 17.0374) -> (-4.1752, 16.7457) centre (-3.9423, 16.8037) ccw
  arc A292 (-3.7386, 14.0189) -> (-3.5676, 14.3088) centre (-3.8005, 14.2508) ccw
  line L149 (-3.5676, 14.3088) -> (-4.1752, 16.7457)
  arc A293 (-4.0648, 14.1756) -> (-3.7717, 14.01) centre (-3.8341, 14.2418) ccw
  arc A294 (-3.7386, 14.0189) -> (-3.7717, 14.01) centre (0, 0) ccw
  line L150 (0, 0) -> (-3.6385, 17.1176) construction
  line L151 (-3.5882, 16.8812) -> (-3.0642, 14.416)
  arc A295 (-4.757, 16.5898) -> (-5.0571, 16.7534) centre (-4.9877, 16.5236) ccw
  arc A296 (-5.0571, 16.7534) -> (-5.1758, 16.7171) centre (0, 0) ccw
  arc A297 (-5.1758, 16.7171) -> (-5.3331, 16.4136) centre (-5.1049, 16.4878) ccw
  arc A298 (-4.7074, 13.7239) -> (-4.557, 14.0251) centre (-4.7853, 13.951) ccw
  line L152 (-4.557, 14.0251) -> (-5.3331, 16.4136)
  arc A299 (-5.0437, 13.8575) -> (-4.7398, 13.7128) centre (-4.8182, 13.9396) ccw
  arc A300 (-4.7074, 13.7239) -> (-4.7398, 13.7128) centre (0, 0) ccw
  line L153 (0, 0) -> (-4.8237, 16.8221) construction
  line L154 (-4.757, 16.5898) -> (-4.0624, 14.1671)
  arc A301 (-5.9027, 16.2175) -> (-6.2134, 16.3598) centre (-6.1282, 16.1354) ccw
  arc A302 (-6.2134, 16.3598) -> (-6.3294, 16.3153) centre (0, 0) ccw
  arc A303 (-6.3294, 16.3153) -> (-6.4651, 16.0016) centre (-6.2426, 16.0916) ccw
  arc A304 (-5.6533, 13.3621) -> (-5.5243, 13.6731) centre (-5.7468, 13.5832) ccw
  line L155 (-5.5243, 13.6731) -> (-6.4651, 16.0016)
  arc A305 (-5.9981, 13.472) -> (-5.6848, 13.3488) centre (-5.7788, 13.5696) ccw
  arc A306 (-5.6533, 13.3621) -> (-5.6848, 13.3488) centre (0, 0) ccw
  line L156 (0, 0) -> (-5.9854, 16.4446) construction
  line L157 (-5.9027, 16.2175) -> (-5.0407, 13.8492)
  arc A307 (-7.0196, 15.7663) -> (-7.3395, 15.8865) centre (-7.2388, 15.6687) ccw
  arc A308 (-7.3395, 15.8865) -> (-7.452, 15.834) centre (0, 0) ccw
  arc A309 (-7.452, 15.834) -> (-7.5656, 15.5117) centre (-7.3498, 15.6169) ccw
  arc A310 (-6.5716, 12.9352) -> (-6.4646, 13.2544) centre (-6.6803, 13.1492) ccw
  line L158 (-6.4646, 13.2544) -> (-7.5656, 15.5117)
  arc A311 (-6.9232, 13.0207) -> (-6.6021, 12.9197) centre (-6.7113, 13.1334) ccw
  arc A312 (-6.5716, 12.9352) -> (-6.6021, 12.9197) centre (0, 0) ccw
  line L159 (0, 0) -> (-7.1179, 15.987) construction
  line L160 (-7.0196, 15.7663) -> (-5.9945, 13.4639)
  arc A313 (-8.1023, 15.2382) -> (-8.4298, 15.3358) centre (-8.3142, 15.1255) ccw
  arc A314 (-8.4298, 15.3358) -> (-8.5384, 15.2756) centre (0, 0) ccw
  arc A315 (-8.5384, 15.2756) -> (-8.6292, 14.9462) centre (-8.4213, 15.0662) ccw
  arc A316 (-7.4579, 12.4453) -> (-7.3734, 12.7712) centre (-7.5813, 12.6512) ccw
  line L161 (-7.3734, 12.7712) -> (-8.6292, 14.9462)
  arc A317 (-7.8147, 12.5061) -> (-7.4873, 12.4277) centre (-7.6111, 12.6332) ccw
  arc A318 (-7.4579, 12.4453) -> (-7.4873, 12.4277) centre (0, 0) ccw
  line L162 (0, 0) -> (-8.2158, 15.4516) construction
  line L163 (-8.1023, 15.2382) -> (-6.9191, 13.0129)
  arc A319 (-9.1455, 14.6359) -> (-9.4791, 14.7105) centre (-9.3491, 14.5087) ccw
  arc A320 (-9.4791, 14.7105) -> (-9.5832, 14.6428) centre (0, 0) ccw
  arc A321 (-9.5832, 14.6428) -> (-9.6507, 14.3078) centre (-9.4518, 14.442) ccw
  arc A322 (-8.3079, 11.8948) -> (-8.2464, 12.2257) centre (-8.4453, 12.0915) ccw
  line L164 (-8.2464, 12.2257) -> (-9.6507, 14.3078)
  arc A323 (-8.668, 11.9305) -> (-8.3359, 11.8751) centre (-8.4738, 12.0715) ccw
  arc A324 (-8.3079, 11.8948) -> (-8.3359, 11.8751) centre (0, 0) ccw
  line L165 (0, 0) -> (-9.2736, 14.8408) construction
  line L166 (-9.1455, 14.6359) -> (-7.81, 12.4986)
  arc A325 (-10.1442, 13.9623) -> (-10.4821, 14.0134) centre (-10.3384, 13.8212) ccw
  arc A326 (-10.4821, 14.0134) -> (-10.5813, 13.9387) centre (0, 0) ccw
  arc A327 (-10.5813, 13.9387) -> (-10.6253, 13.5998) centre (-10.4362, 13.7475) ccw
  arc A328 (-9.1174, 11.2863) -> (-9.0791, 11.6207) centre (-9.2682, 11.4729) ccw
  line L167 (-9.0791, 11.6207) -> (-10.6253, 13.5998)
  arc A329 (-9.4791, 11.2968) -> (-9.144, 11.2647) centre (-9.2953, 11.451) ccw
  arc A330 (-9.1174, 11.2863) -> (-9.144, 11.2647) centre (0, 0) ccw
  line L168 (0, 0) -> (-10.2862, 14.1578) construction
  line L169 (-10.1442, 13.9623) -> (-8.6628, 11.9233)
  arc A331 (-11.0934, 13.2206) -> (-11.4341, 13.2481) centre (-11.2773, 13.0664) ccw
  arc A332 (-11.4341, 13.2481) -> (-11.5278, 13.1666) centre (0, 0) ccw
  arc A333 (-11.5278, 13.1666) -> (-11.5481, 12.8254) centre (-11.3697, 12.986) ccw
  arc A334 (-9.8825, 10.6228) -> (-9.8676, 10.9591) centre (-10.0459, 10.7985) ccw
  line L170 (-9.8676, 10.9591) -> (-11.5481, 12.8254)
  arc A335 (-10.244, 10.608) -> (-9.9075, 10.5994) centre (-10.0714, 10.7747) ccw
  arc A336 (-9.8825, 10.6228) -> (-9.9075, 10.5994) centre (0, 0) ccw
  line L171 (0, 0) -> (-11.2488, 13.4058) construction
  line L172 (-11.0934, 13.2206) -> (-9.4734, 11.29)
  arc A337 (-11.9886, 12.4146) -> (-12.3304, 12.4182) centre (-12.1613, 12.2479) ccw
  arc A338 (-12.3304, 12.4182) -> (-12.4182, 12.3304) centre (0, 0) ccw
  arc A339 (-12.4182, 12.3304) -> (-12.4146, 11.9886) centre (-12.2479, 12.1613) ccw
  arc A340 (-10.5994, 9.9075) -> (-10.608, 10.244) centre (-10.7747, 10.0714) ccw
  line L173 (-10.608, 10.244) -> (-12.4146, 11.9886)
  arc A341 (-10.9591, 9.8676) -> (-10.6228, 9.8825) centre (-10.7985, 10.0459) ccw
  arc A342 (-10.5994, 9.9075) -> (-10.6228, 9.8825) centre (0, 0) ccw
  line L174 (0, 0) -> (-12.1565, 12.5884) construction
  line L175 (-11.9886, 12.4146) -> (-10.2379, 10.6017)
  arc A343 (-12.8254, 11.5481) -> (-13.1666, 11.5278) centre (-12.986, 11.3697) ccw
  arc A344 (-13.1666, 11.5278) -> (-13.2481, 11.4341) centre (0, 0) ccw
  arc A345 (-13.2481, 11.4341) -> (-13.2206, 11.0934) centre (-13.0664, 11.2773) ccw
  arc A346 (-11.2647, 9.144) -> (-11.2968, 9.4791) centre (-11.451, 9.2953) ccw
  line L176 (-11.2968, 9.4791) -> (-13.2206, 11.0934)
  arc A347 (-11.6207, 9.0791) -> (-11.2863, 9.1174) centre (-11.4729, 9.2682) ccw
  arc A348 (-11.2647, 9.144) -> (-11.2863, 9.1174) centre (0, 0) ccw
  line L177 (0, 0) -> (-13.005, 11.7098) construction
  line L178 (-12.8254, 11.5481) -> (-10.9525, 9.8617)
  arc A349 (-13.5998, 10.6253) -> (-13.9387, 10.5813) centre (-13.7475, 10.4362) ccw
  arc A350 (-13.9387, 10.5813) -> (-14.0134, 10.4821) centre (0, 0) ccw
  arc A351 (-14.0134, 10.4821) -> (-13.9623, 10.1442) centre (-13.8212, 10.3384) ccw
  arc A352 (-11.8751, 8.3359) -> (-11.9305, 8.668) centre (-12.0715, 8.4738) ccw
  line L179 (-11.9305, 8.668) -> (-13.9623, 10.1442)
  arc A353 (-12.2257, 8.2464) -> (-11.8948, 8.3079) centre (-12.0915, 8.4453) ccw
  arc A354 (-11.8751, 8.3359) -> (-11.8948, 8.3079) centre (0, 0) ccw
  line L180 (0, 0) -> (-13.7902, 10.7741) construction
  line L181 (-13.5998, 10.6253) -> (-11.6137, 9.0736)
  arc A355 (-14.3078, 9.6507) -> (-14.6428, 9.5832) centre (-14.442, 9.4518) ccw
  arc A356 (-14.6428, 9.5832) -> (-14.7105, 9.4791) centre (0, 0) ccw
  arc A357 (-14.7105, 9.4791) -> (-14.6359, 9.1455) centre (-14.5087, 9.3491) ccw
  arc A358 (-12.4277, 7.4873) -> (-12.5061, 7.8147) centre (-12.6332, 7.6111) ccw
  line L182 (-12.5061, 7.8147) -> (-14.6359, 9.1455)
  arc A359 (-12.7712, 7.3734) -> (-12.4453, 7.4579) centre (-12.6512, 7.5813) ccw
  arc A360 (-12.4277, 7.4873) -> (-12.4453, 7.4579) centre (0, 0) ccw
  line L183 (0, 0) -> (-14.5082, 9.7859) construction
  line L184 (-14.3078, 9.6507) -> (-12.2184, 8.2414)
  arc A361 (-14.9462, 8.6292) -> (-15.2756, 8.5384) centre (-15.0662, 8.4213) ccw
  arc A362 (-15.2756, 8.5384) -> (-15.3358, 8.4298) centre (0, 0) ccw
  arc A363 (-15.3358, 8.4298) -> (-15.2382, 8.1023) centre (-15.1255, 8.3142) ccw
  arc A364 (-12.9197, 6.6021) -> (-13.0207, 6.9232) centre (-13.1334, 6.7113) ccw
  line L185 (-13.0207, 6.9232) -> (-15.2382, 8.1023)
  arc A365 (-13.2544, 6.4646) -> (-12.9352, 6.5716) centre (-13.1492, 6.6803) ccw
  arc A366 (-12.9197, 6.6021) -> (-12.9352, 6.5716) centre (0, 0) ccw
  line L186 (0, 0) -> (-15.1554, 8.75) construction
  line L187 (-14.9462, 8.6292) -> (-12.7635, 7.369)
  arc A367 (-15.5117, 7.5656) -> (-15.834, 7.452) centre (-15.6169, 7.3498) ccw
  arc A368 (-15.834, 7.452) -> (-15.8865, 7.3395) centre (0, 0) ccw
  arc A369 (-15.8865, 7.3395) -> (-15.7663, 7.0196) centre (-15.6687, 7.2388) ccw
  arc A370 (-13.3488, 5.6848) -> (-13.472, 5.9981) centre (-13.5696, 5.7788) ccw
  line L188 (-13.472, 5.9981) -> (-15.7663, 7.0196)
  arc A371 (-13.6731, 5.5243) -> (-13.3621, 5.6533) centre (-13.5832, 5.7468) ccw
  arc A372 (-13.3488, 5.6848) -> (-13.3621, 5.6533) centre (0, 0) ccw
  line L189 (0, 0) -> (-15.7289, 7.6715) construction
  line L190 (-15.5117, 7.5656) -> (-13.2465, 6.4607)
  arc A373 (-16.0016, 6.4651) -> (-16.3153, 6.3294) centre (-16.0916, 6.2426) ccw
  arc A374 (-16.3153, 6.3294) -> (-16.3598, 6.2134) centre (0, 0) ccw
  arc A375 (-16.3598, 6.2134) -> (-16.2175, 5.9027) centre (-16.1354, 6.1282) ccw
  arc A376 (-13.7128, 4.7398) -> (-13.8575, 5.0437) centre (-13.9396, 4.8182) ccw
  line L191 (-13.8575, 5.0437) -> (-16.2175, 5.9027)
  arc A377 (-14.0251, 4.557) -> (-13.7239, 4.7074) centre (-13.951, 4.7853) ccw
  arc A378 (-13.7128, 4.7398) -> (-13.7239, 4.7074) centre (0, 0) ccw
  line L192 (0, 0) -> (-16.2257, 6.5556) construction
  line L193 (-16.0016, 6.4651) -> (-13.6649, 5.521)
  arc A379 (-16.4136, 5.3331) -> (-16.7171, 5.1758) centre (-16.4878, 5.1049) ccw
  arc A380 (-16.7171, 5.1758) -> (-16.7534, 5.0571) centre (0, 0) ccw
  arc A381 (-16.7534, 5.0571) -> (-16.5898, 4.757) centre (-16.5236, 4.9877) ccw
  arc A382 (-14.01, 3.7717) -> (-14.1756, 4.0648) centre (-14.2418, 3.8341) ccw
  line L194 (-14.1756, 4.0648) -> (-16.5898, 4.757)
  arc A383 (-14.3088, 3.5676) -> (-14.0189, 3.7386) centre (-14.2508, 3.8005) ccw
  arc A384 (-14.01, 3.7717) -> (-14.0189, 3.7386) centre (0, 0) ccw
  line L195 (0, 0) -> (-16.6435, 5.4078) construction
  line L196 (-16.4136, 5.3331) -> (-14.0167, 4.5543)
  arc A385 (-16.7457, 4.1752) -> (-17.0374, 3.9971) centre (-16.8037, 3.9423) ccw
  arc A386 (-17.0374, 3.9971) -> (-17.0653, 3.8761) centre (0, 0) ccw
  arc A387 (-17.0653, 3.8761) -> (-16.8812, 3.5882) centre (-16.8313, 3.823) ccw
  arc A388 (-14.239, 2.7852) -> (-14.4246, 3.066) centre (-14.4745, 2.8313) ccw
  line L197 (-14.4246, 3.066) -> (-16.8812, 3.5882)
  arc A389 (-14.5228, 2.5608) -> (-14.2455, 2.7516) centre (-14.4812, 2.7971) ccw
  arc A390 (-14.239, 2.7852) -> (-14.2455, 2.7516) centre (0, 0) ccw
  line L198 (0, 0) -> (-16.9802, 4.2336) construction
  line L199 (-16.7457, 4.1752) -> (-14.3003, 3.5655)
  arc A391 (-16.9961, 2.9969) -> (-17.2747, 2.7989) centre (-17.0378, 2.7605) ccw
  arc A392 (-17.2747, 2.7989) -> (-17.2941, 2.6763) centre (0, 0) ccw
  arc A393 (-17.2941, 2.6763) -> (-17.0904, 2.4019) centre (-17.057, 2.6396) ccw
  arc A394 (-14.3986, 1.7852) -> (-14.6034, 2.0524) centre (-14.6368, 1.8147) ccw
  line L200 (-14.6034, 2.0524) -> (-17.0904, 2.4019)
  arc A395 (-14.6661, 1.5415) -> (-14.4028, 1.7512) centre (-14.641, 1.7802) ccw
  arc A396 (-14.3986, 1.7852) -> (-14.4028, 1.7512) centre (0, 0) ccw
  line L201 (0, 0) -> (-17.2341, 3.0388) construction
  line L202 (-16.9961, 2.9969) -> (-14.5141, 2.5592)
  arc A397 (-17.1638, 1.804) -> (-17.4279, 1.5871) centre (-17.1889, 1.5653) ccw
  arc A398 (-17.4279, 1.5871) -> (-17.4387, 1.4634) centre (0, 0) ccw
  arc A399 (-17.4387, 1.4634) -> (-17.2163, 1.2039) centre (-17.1995, 1.4433) ccw
  arc A400 (-14.488, 0.7764) -> (-14.711, 1.0287) centre (-14.7277, 0.7893) ccw
  line L203 (-14.711, 1.0287) -> (-17.2163, 1.2039)
  arc A401 (-14.7379, 0.5147) -> (-14.4898, 0.7422) centre (-14.7295, 0.7545) ccw
  arc A402 (-14.488, 0.7764) -> (-14.4898, 0.7422) centre (0, 0) ccw
  line L204 (0, 0) -> (-17.4041, 1.8292) construction
  line L205 (-17.1638, 1.804) -> (-14.6573, 1.5405)
  arc A403 (-17.2478, 0.6023) -> (-17.4961, 0.3675) centre (-17.2562, 0.3625) ccw
  arc A404 (-17.4961, 0.3675) -> (-17.4983, 0.2433) centre (0, 0) ccw
  arc A405 (-17.4983, 0.2433) -> (-17.2583, 0) centre (-17.2583, 0.24) ccw
  arc A406 (-14.5069, -0.2361) -> (-14.7469, 0) centre (-14.7469, -0.24) ccw
  line L206 (-14.7469, 0) -> (-17.2583, 0)
  arc A407 (-14.7379, -0.5147) -> (-14.5063, -0.2703) centre (-14.7463, -0.2748) ccw
  arc A408 (-14.5069, -0.2361) -> (-14.5063, -0.2703) centre (0, 0) ccw
  line L207 (0, 0) -> (-17.4893, 0.6107) construction
  line L208 (-17.2478, 0.6023) -> (-14.7291, 0.5144)
  arc A409 (-17.2478, -0.6023) -> (-17.4792, -0.8539) centre (-17.2394, -0.8422) ccw
  arc A410 (-17.4792, -0.8539) -> (-17.4727, -0.9779) centre (0, 0) ccw
  arc A411 (-17.4727, -0.9779) -> (-17.2163, -1.2039) centre (-17.233, -0.9645) ccw
  arc A412 (-14.4551, -1.2475) -> (-14.711, -1.0287) centre (-14.6942, -1.2681) ccw
  line L209 (-14.711, -1.0287) -> (-17.2163, -1.2039)
  arc A413 (-14.6661, -1.5415) -> (-14.4521, -1.2816) centre (-14.6912, -1.3028) ccw
  arc A414 (-14.4551, -1.2475) -> (-14.4521, -1.2816) centre (0, 0) ccw
  line L210 (0, 0) -> (-17.4893, -0.6107) construction
  line L211 (-17.2478, -0.6023) -> (-14.7291, -0.5144)
  arc A415 (-17.1638, -1.804) -> (-17.377, -2.0711) centre (-17.1387, -2.0427) ccw
  arc A416 (-17.377, -2.0711) -> (-17.3619, -2.1943) centre (0, 0) ccw
  arc A417 (-17.3619, -2.1943) -> (-17.0904, -2.4019) centre (-17.1238, -2.1642) ccw
  arc A418 (-14.3329, -2.2528) -> (-14.6034, -2.0524) centre (-14.57, -2.29) ccw
  line L212 (-14.6034, -2.0524) -> (-17.0904, -2.4019)
  arc A419 (-14.5228, -2.5608) -> (-14.3275, -2.2866) centre (-14.5645, -2.3244) ccw
  arc A420 (-14.3329, -2.2528) -> (-14.3275, -2.2866) centre (0, 0) ccw
  line L213 (0, 0) -> (-17.4041, -1.8292) construction
  line L214 (-17.1638, -1.804) -> (-14.6573, -1.5405)
  arc A421 (-16.9961, -2.9969) -> (-17.1902, -3.2782) centre (-16.9545, -3.2332) ccw
  arc A422 (-17.1902, -3.2782) -> (-17.1665, -3.4001) centre (0, 0) ccw
  arc A423 (-17.1665, -3.4001) -> (-16.8812, -3.5882) centre (-16.9311, -3.3535) ccw
  arc A424 (-14.1408, -3.2471) -> (-14.4246, -3.066) centre (-14.3747, -3.3008) ccw
  line L215 (-14.4246, -3.066) -> (-16.8812, -3.5882)
  arc A425 (-14.3088, -3.5676) -> (-14.1331, -3.2805) centre (-14.3669, -3.3347) ccw
  arc A426 (-14.1408, -3.2471) -> (-14.1331, -3.2805) centre (0, 0) ccw
  line L216 (0, 0) -> (-17.2341, -3.0388) construction
  line L217 (-16.9961, -2.9969) -> (-14.5141, -2.5592)
  arc A427 (-16.7457, -4.1752) -> (-16.9197, -4.4693) centre (-16.6876, -4.408) ccw
  arc A428 (-16.9197, -4.4693) -> (-16.8875, -4.5893) centre (0, 0) ccw
  arc A429 (-16.8875, -4.5893) -> (-16.5898, -4.757) centre (-16.6559, -4.5263) ccw
  arc A430 (-13.8799, -4.2256) -> (-14.1756, -4.0648) centre (-14.1095, -4.2955) ccw
  line L218 (-14.1756, -4.0648) -> (-16.5898, -4.757)
  arc A431 (-14.0251, -4.557) -> (-13.8699, -4.2583) centre (-14.0993, -4.3288) ccw
  arc A432 (-13.8799, -4.2256) -> (-13.8699, -4.2583) centre (0, 0) ccw
  line L219 (0, 0) -> (-16.9802, -4.2336) construction
  line L220 (-16.7457, -4.1752) -> (-14.3003, -3.5655)
  arc A433 (-16.4136, -5.3331) -> (-16.5667, -5.6387) centre (-16.3395, -5.5614) ccw
  arc A434 (-16.5667, -5.6387) -> (-16.5263, -5.7561) centre (0, 0) ccw
  arc A435 (-16.5263, -5.7561) -> (-16.2175, -5.9027) centre (-16.2996, -5.6772) ccw
  arc A436 (-13.5513, -5.1835) -> (-13.8575, -5.0437) centre (-13.7755, -5.2693) ccw
  line L221 (-13.8575, -5.0437) -> (-16.2175, -5.9027)
  arc A437 (-13.6731, -5.5243) -> (-13.539, -5.2155) centre (-13.763, -5.3018) ccw
  arc A438 (-13.5513, -5.1835) -> (-13.539, -5.2155) centre (0, 0) ccw
  line L222 (0, 0) -> (-16.6435, -5.4078) construction
  line L223 (-16.4136, -5.3331) -> (-14.0167, -4.5543)
  arc A439 (-16.0016, -6.4651) -> (-16.133, -6.7806) centre (-15.9117, -6.6876) ccw
  arc A440 (-16.133, -6.7806) -> (-16.0845, -6.8949) centre (0, 0) ccw
  arc A441 (-16.0845, -6.8949) -> (-15.7663, -7.0196) centre (-15.8639, -6.8003) ccw
  arc A442 (-13.1567, -6.1162) -> (-13.472, -5.9981) centre (-13.3743, -6.2173) ccw
  line L224 (-13.472, -5.9981) -> (-15.7663, -7.0196)
  arc A443 (-13.2544, -6.4646) -> (-13.1422, -6.1472) centre (-13.3596, -6.2489) ccw
  arc A444 (-13.1567, -6.1162) -> (-13.1422, -6.1472) centre (0, 0) ccw
  line L225 (0, 0) -> (-16.2257, -6.5556) construction
  line L226 (-16.0016, -6.4651) -> (-13.6649, -5.521)
  arc A445 (-15.5117, -7.5656) -> (-15.6207, -7.8895) centre (-15.4065, -7.7813) ccw
  arc A446 (-15.6207, -7.8895) -> (-15.5643, -8.0001) centre (0, 0) ccw
  arc A447 (-15.5643, -8.0001) -> (-15.2382, -8.1023) centre (-15.3509, -7.8904) ccw
  arc A448 (-12.698, -7.019) -> (-13.0207, -6.9232) centre (-12.9081, -7.1352) ccw
  line L227 (-13.0207, -6.9232) -> (-15.2382, -8.1023)
  arc A449 (-12.7712, -7.3734) -> (-12.6814, -7.049) centre (-12.8912, -7.1656) ccw
  arc A450 (-12.698, -7.019) -> (-12.6814, -7.049) centre (0, 0) ccw
  line L228 (0, 0) -> (-15.7289, -7.6715) construction
  line L229 (-15.5117, -7.5656) -> (-13.2465, -6.4607)
  arc A451 (-14.9462, -8.6292) -> (-15.0323, -8.9599) centre (-14.8262, -8.837) ccw
  arc A452 (-15.0323, -8.9599) -> (-14.9684, -9.0663) centre (0, 0) ccw
  arc A453 (-14.9684, -9.0663) -> (-14.6359, -9.1455) centre (-14.7631, -8.942) ccw
  arc A454 (-12.1775, -7.8877) -> (-12.5061, -7.8147) centre (-12.3789, -8.0182) ccw
  line L230 (-12.5061, -7.8147) -> (-14.6359, -9.1455)
  arc A455 (-12.2257, -8.2464) -> (-12.1588, -7.9164) centre (-12.3599, -8.0474) ccw
  arc A456 (-12.1775, -7.8877) -> (-12.1588, -7.9164) centre (0, 0) ccw
  line L231 (0, 0) -> (-15.1554, -8.75) construction
  line L232 (-14.9462, -8.6292) -> (-12.7635, -7.369)
  arc A457 (-14.3078, -9.6507) -> (-14.3707, -9.9867) centre (-14.1736, -9.8497) ccw
  arc A458 (-14.3707, -9.9867) -> (-14.2995, -10.0884) centre (0, 0) ccw
  arc A459 (-14.2995, -10.0884) -> (-13.9623, -10.1442) centre (-14.1034, -9.95) ccw